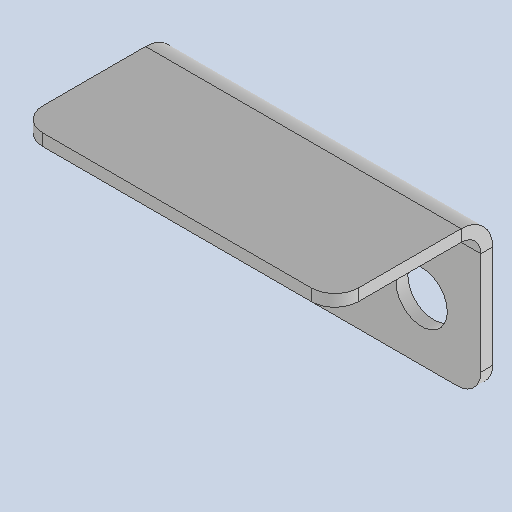
# Autodesk Inventor part: MSC 912 flange slipway
Saved by Autodesk Inventor 2025 (Build 290162010, 162A)
## iProperties
Created: 2024-07-01
Part Number: MSC 912 flange slipway
Material: Stainless Steel
Document SubType Name: Sheet Metal
Designer: admin
Stock Number: МОО 902 опора рамы
Mass: 135.371 g
Surface Area: 124.203 cm^2
Volume: 16.9213 cm^3
Density: 8 g/cm^3
Sheet Metal Rule: AISI304 3mm Die 32
Sheet Metal Width: 73,927 mm
Sheet Metal Length: 80,000 mm
Sheet Metal Area: 5914,195 mm^2
Appearance: Default
Flat Pattern Width: 7.39274 cm
Flat Pattern Length: 8 cm
Flat Pattern Area: 59.1419 cm^2
Author: pokla
Autodesk Inventor part; units mm, degrees
ref_plane "YZ Plane" through (0, 0, 0) normal (1, 0, 0) x (0, 1, 0)
ref_plane "XZ Plane" through (0, 0, 0) normal (0, 1, 0) x (-1, 0, 0)
ref_plane "XY Plane" through (0, 0, 0) normal (0, 0, 1) x (1, 0, 0)
sketch "Sketch4" plane through (0, 0, 0) normal (0, 1, 0) x (-1, 0, 0)
  line L0 (40, -40) -> (-40, -40)
  line L1 (-40, -40) -> (-40, 0)
  line L2 (-40, 0) -> (40, 0)
  line L3 (40, 0) -> (40, -40)
  point P0 (0, 0)
  point P1 (0, 0)
  dimension "d36" = 80
  dimension "d37" = 40
  measures "d36" distance of L0.start L0.end
  measures "d37" distance between parallel lines of L0 L2
extrude "Plate2" add sketch "Sketch4" along normal blind 3
sketch "Sketch5" plane through (0, 0, 0) normal (0, -1, 0) x (1, 0, 0)
  circle A0 centre (-25, -25) radius 6.5
  circle A1 centre (25, -25) radius 6.5
  line L0 (0, 0) -> (0, -40) construction
  line L1 (40, -40) -> (-40, -40) construction
  dimension "d39" = 50
  dimension "d40" = 15
  dimension "d41" = 13
  constraints: 2 centre point, 2 end point, 1 midpoint, 1 other
  measures "d39" distance of A1.centre A0.centre
  measures "d40" distance from line of L1 A1.centre
  measures "d41" diameter of A1
extrude "Cut1" cut sketch "Sketch5" against normal blind 3
sketch "Sketch6" plane through (-40, 3, -3) normal (0, 0, 1) x (1, 0, 0)
  line L0 (80, 0) -> (0, 0)
  line L1 (0, 0) -> (0, -40)
  line L2 (0, -40) -> (80, -40)
  line L3 (80, -40) -> (80, 0)
  constraints: 6 end point, 1 horizontal, 1 perpendicular, 1 vertical
edge flange "Flange1" height 40 angle 90 thickness 3 bend radius 5 thickness toward (0, 0, 1) relief round relief width 3 relief depth 1.5 edges at (0, 0, 0) wall of the first edge with corners at (40, 3, -3) (-40, 3, -3) (-40, -37, -3) (40, -37, -3)
bend "Bend1"
corner "Corner1"
fillet "Corner Round6" radius 6 4 edges at (40, -37, -1.5) (-40, 1.5, -40) (40, 1.5, -40) (-40, -37, -1.5)
equation "\"d42\" = Thickness"
equation "\"d38\" = Thickness"
equation "\"d44\" = BendReliefWidth"
equation "\"d45\" = BendReliefDepth"
equation "\"d46\" = MinimumRemnant"
equation "\"d47\" = TransitionRadius"
equation "\"d50\" = BendRadius"
equation "\"d51\" = CornerReliefSize"
equation "\"d52\" = GapSize"
equation "\"d53\" = JacobiRadiusSize"
equation "\"BendReliefWidth\" = Thickness"
equation "\"BendReliefDepth\" = 0.5 * Thickness"
equation "\"CornerReliefSize\" = 4 * Thickness"
equation "\"MinimumRemnant\" = 2 * Thickness"
equation "\"TransitionRadius\" = BendRadius"
equation "\"JacobiRadiusSize\" = BendRadius"
equation "\"GapSize\" = Thickness"
equation "\"Thickness\" = 3"
equation "\"BendRadius\" = 5"
body "Solid2"
